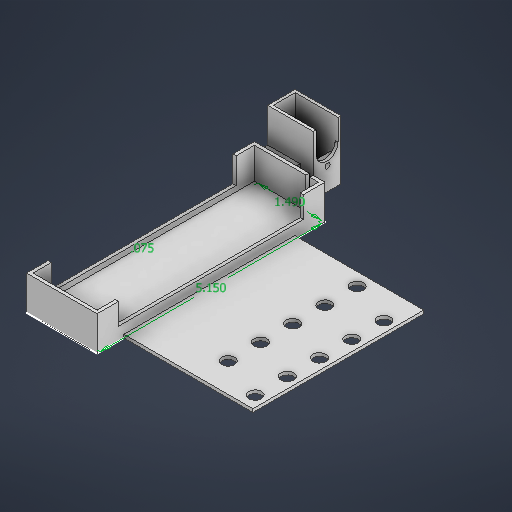
# Autodesk Inventor part: HarmonicaFrame2
Saved by Autodesk Inventor 2026.2 (Build 302298010, 298A)
## iProperties
Created: 2026-03-08
Part Number: HarmonicaFrame2
Material: Generic
Document SubType Name: Modeling
Designer: david
Density: 1 g/cm^3
Appearance: Default
Author: david
Autodesk Inventor part; units mm, degrees
ref_plane "YZ Plane" through (0, 0, 0) normal (1, 0, 0) x (0, 1, 0)
ref_plane "XZ Plane" through (0, 0, 0) normal (0, 1, 0) x (-1, 0, 0)
ref_plane "XY Plane" through (0, 0, 0) normal (0, 0, 1) x (1, 0, 0)
sketch "Sketch1" plane through (0, 0, 0) normal (0, 1, 0) x (-1, 0, 0)
  line L0 (18.923, 65.405) -> (-18.923, 65.405)
  line L1 (-18.923, 65.405) -> (-18.923, -65.405)
  line L2 (-18.923, -65.405) -> (18.923, -65.405)
  line L3 (18.923, -65.405) -> (18.923, 65.405)
  line L4 (18.923, 65.405) -> (-18.923, -65.405) construction
  line L5 (-18.923, 65.405) -> (18.923, -65.405) construction
  line L6 (20.828, 67.31) -> (-20.828, 67.31)
  line L7 (-20.828, 67.31) -> (-20.828, -67.31)
  line L8 (-20.828, -67.31) -> (20.828, -67.31)
  line L9 (20.828, -67.31) -> (20.828, 67.31)
  point P0 (0, 0)
  dimension "d0" = 37.846
  dimension "d1" = 130.81
  dimension "d2" = 1.905
  constraints: 20 end point, 4 parallel, 2 midpoint, 2 perpendicular, 1 horizontal, 3 other
  measures "d0" distance of L2.end L1.end
  measures "d1" distance of L1.end L0.end
  measures "d2" distance between parallel lines of L3 L9
extrude "Extrusion1" add sketch "Sketch1" along normal blind 20.32
extrude "Extrusion2" add sketch "Sketch1" along normal blind 1.905 contours L3 L2 L1 L0
sketch "Sketch2" plane through (20.828, 0, 67.31) normal (1, 0, 0) x (0, 0, -1)
  line L0 (12.7, 20.32) -> (121.92, 20.32)
  line L1 (121.92, 20.32) -> (121.92, 7.62)
  line L2 (121.92, 7.62) -> (12.7, 7.62)
  line L3 (12.7, 7.62) -> (12.7, 20.32)
  line L4 (0, 0) -> (0, 20.32) projected
  line L5 (134.62, 0) -> (134.62, 20.32) projected
  line L6 (0, 20.32) -> (134.62, 20.32) projected
  line L7 (0, 0) -> (134.62, 0) projected
  point P0 (67.31, 0)
  dimension "d7" = 12.7
  dimension "d8" = 12.7
  dimension "d9" = 7.62
  constraints: 8 end point, 2 parallel, 1 collinear, 1 horizontal, 1 perpendicular
  measures "d7" distance between parallel lines of L4 L3
  measures "d8" distance between parallel lines of L5 L1
  measures "d9" distance between parallel lines of L7 L2
extrude "Extrusion3" cut sketch "Sketch2" against normal blind 1.905 contours L0 L1 L2 L3
sketch "Sketch3" plane through (-20.828, 0, -67.31) normal (-1, 0, 0) x (0, 0, 1)
  line L0 (12.7, 20.32) -> (121.92, 20.32)
  line L1 (121.92, 20.32) -> (121.92, 5.08)
  line L2 (121.92, 5.08) -> (12.7, 5.08)
  line L3 (12.7, 5.08) -> (12.7, 20.32)
  line L4 (0, 20.32) -> (134.62, 20.32) projected
  line L5 (0, 0) -> (0, 20.32) projected
  line L6 (134.62, 0) -> (134.62, 20.32) projected
  line L7 (0, 0) -> (134.62, 0) projected
  point P0 (67.31, 0)
  dimension "d12" = 12.7
  dimension "d13" = 12.7
  dimension "d14" = 5.08
  constraints: 8 end point, 2 parallel, 1 collinear, 1 horizontal, 1 perpendicular
  measures "d12" distance between parallel lines of L5 L3
  measures "d13" distance between parallel lines of L6 L1
  measures "d14" distance between parallel lines of L7 L2
extrude "Extrusion4" cut sketch "Sketch3" against normal blind 1.905 contours L0 L1 L2 L3
sketch "Sketch4" plane through (0, 20.32, 0) normal (0, 1, 0) x (1, 0, 0)
  line L0 (20.828, 67.31) -> (-20.828, 67.31) projected
  line L1 (-18.923, 65.405) -> (18.923, 65.405) projected
  line L2 (13.843, 67.31) -> (11.557, 67.31)
  line L3 (11.557, 67.31) -> (11.557, 65.405)
  line L4 (11.557, 65.405) -> (13.843, 65.405)
  line L5 (13.843, 65.405) -> (13.843, 67.31)
  line L6 (18.923, 65.405) -> (18.923, 54.61) projected
  line L7 (-18.923, 54.61) -> (-18.923, 65.405) projected
  point P0 (0, 0)
  dimension "d17" = 5.08
  dimension "d18" = 30.48
  constraints: 8 end point, 2 parallel, 2 point on line, 1 horizontal, 1 perpendicular
  measures "d17" distance between parallel lines of L6 L5
  measures "d18" distance between parallel lines of L7 L3
extrude "Extrusion5" cut sketch "Sketch4" against normal up to surface (18.415 mm away)
sketch "Sketch5" plane through (20.828, 0, -67.31) normal (0, 0, -1) x (-1, 0, 0)
  line L0 (0, 0) -> (41.656, 0) projected
  line L1 (0, 0) -> (41.656, 0)
  line L2 (41.656, 0) -> (41.656, 1.905)
  line L3 (41.656, 1.905) -> (0, 1.905)
  line L4 (0, 1.905) -> (0, 0)
  line L5 (9.271, 1.905) -> (6.985, 1.905) projected
  line L6 (41.656, 0) -> (41.656, 20.32) projected
  point P0 (20.828, 0)
  constraints: 8 end point, 2 collinear, 2 parallel, 1 horizontal, 1 perpendicular
extrude "Extrusion6" add sketch "Sketch5" along normal blind 24.13
sketch "Sketch6" plane through (0, 1.905, 0) normal (0, 1, 0) x (1, 0, 0)
  line L0 (-19.177, 76.835) -> (4.445, 76.835)
  line L1 (4.445, 76.835) -> (4.445, 89.789)
  line L2 (4.445, 89.789) -> (-19.177, 89.789)
  line L3 (-19.177, 89.789) -> (-19.177, 76.835)
  line L4 (18.923, 65.405) -> (18.923, 54.61) projected
  line L5 (11.557, 67.31) -> (-20.828, 67.31) projected
  line L6 (-20.828, 75.184) -> (6.096, 75.184)
  line L7 (6.096, 75.184) -> (6.096, 91.44)
  line L8 (6.096, 91.44) -> (-20.828, 91.44)
  line L9 (-20.828, 91.44) -> (-20.828, 75.184)
  line L10 (-20.828, 91.44) -> (20.828, 91.44) projected
  line L11 (-20.828, 67.31) -> (-20.828, 91.44) projected
  line L12 (-18.923, 65.405) -> (11.557, 65.405) projected
  point P0 (0, 0)
  dimension "d24" = 12.954
  dimension "d26" = 23.622
  dimension "d32" = 11.43
  constraints: 16 end point, 4 parallel, 2 collinear, 2 perpendicular, 1 horizontal, 3 other
  measures "d24" distance between parallel lines of L2 L0
  measures "d26" distance between parallel lines of L1 L3
  measures "d32" distance between parallel lines of L12 L0
extrude "Extrusion7" add sketch "Sketch6" along normal blind 33.02
sketch "Sketch8" plane through (4.445, 1.905, -89.789) normal (-1, 0, 0) x (0, 0, 1)
  circle A0 centre (6.477, 20.32) radius 6.477
  line L0 (0, 0) -> (0, 33.02) projected
  line L1 (12.954, 0) -> (12.954, 33.02) projected
  line L2 (0, 0) -> (12.954, 0) projected
  line L3 (12.954, 20.32) -> (12.954, 33.02)
  line L4 (0, 33.02) -> (0, 20.32)
  line L5 (12.954, 33.02) -> (0, 33.02)
  line L6 (12.954, 20.32) -> (12.954, 33.02)
  line L7 (0, 33.02) -> (0, 20.32)
  point P0 (89.789, -1.905)
  dimension "d29" = 20.32
  constraints: 10 end point, 5 tangent, 2 collinear, 2 point on circle, 2 point on line, 1 centre point, 1 parallel, 1 perpendicular
  measures "d29" distance from line of L2 A0.centre
extrude "Extrusion8" cut sketch "Sketch8" against normal blind 33.02 contours A0 | A0 L0 L5 L1
sketch "Sketch10" plane through (4.445, 1.905, -89.789) normal (-1, 0, 0) x (0, 0, 1)
  line L0 (-1.651, 0) -> (14.605, 0) projected
  line L1 (-1.651, 0) -> (-1.651, 33.02) projected
  line L2 (14.605, 0) -> (-1.651, 0)
  line L3 (-1.651, 0) -> (-1.651, 13.208)
  line L4 (-1.651, 13.208) -> (14.605, 13.208)
  line L5 (14.605, 13.208) -> (14.605, 0)
  arc A0 (0, 20.32) -> (12.954, 20.32) centre (6.477, 20.32) ccw projected
  point P0 (89.789, -1.905)
  point P1 (6.477, 13.843)
  point P2 (6.477, 13.208)
  dimension "d37" = 0.635
  constraints: 8 end point, 2 parallel, 1 horizontal, 1 midpoint, 1 perpendicular, 1 point on circle, 1 point on line
  measures "d37" distance of point (6.477, 13.843) point (6.477, 13.208)
extrude "Extrusion10" add sketch "Sketch10" along normal blind 3.048
sketch "Sketch9" plane through (6.096, 1.905, -75.184) normal (1, 0, 0) x (0, 0, -1)
  arc A0 (1.651, 20.32) -> (14.605, 20.32) centre (8.128, 20.32) ccw projected
  circle A1 centre (8.372, 11.303) radius 1.524
  point P0 (-75.184, -1.905)
  point P1 (8.128, 13.843)
  dimension "d33" = 2.54
  dimension "d34" = 3.048
  constraints: 1 centre point, 1 coincident, 1 point on circle
  measures "d33" vertical distance of point (8.372, 11.303) point (8.128, 13.843)
  measures "d34" diameter of A1
extrude "Extrusion9" cut sketch "Sketch9" against normal up to surface (25.273 mm away)
sketch "Sketch11" plane through (20.828, 0, 67.31) normal (1, 0, 0) x (0, 0, -1)
  line L0 (134.62, 1.905) -> (158.75, 1.905) projected
  line L1 (0, 0) -> (158.75, 0)
  line L2 (158.75, 0) -> (158.75, 1.905)
  line L3 (158.75, 1.905) -> (0, 1.905)
  line L4 (0, 1.905) -> (0, 0)
  point P0 (67.31, 0)
  constraints: 8 end point, 2 parallel, 1 horizontal, 1 perpendicular
extrude "Extrusion11" add sketch "Sketch11" along normal blind 76.2
sketch "Sketch12" plane through (0, 1.905, 0) normal (0, 1, 0) x (1, 0, 0)
  circle A0 centre (90.678, -43.815) radius 3.81
  line L0 (20.828, 54.61) -> (20.828, -54.61) projected
  line L1 (18.923, -65.405) -> (-18.923, -65.405) projected
  line L2 (20.828, -51.435) -> (97.028, -51.435)
  line L3 (97.028, 91.44) -> (97.028, -67.31) projected
  line L4 (97.028, -67.31) -> (20.828, -67.31)
  line L5 (20.828, -67.31) -> (20.828, -51.435)
  line L6 (97.028, -36.195) -> (20.828, -36.195)
  line L7 (-20.828, 91.44) -> (97.028, 91.44) projected
  line L8 (20.828, 91.44) -> (97.028, 91.44)
  line L9 (97.028, 91.44) -> (97.028, -36.195)
  line L10 (20.828, -36.195) -> (97.028, -36.195)
  line L11 (97.028, -36.195) -> (97.028, 91.44)
  line L12 (97.028, 91.44) -> (20.828, 91.44)
  line L13 (20.828, 91.44) -> (20.828, -36.195)
  line L14 (6.096, 91.44) -> (97.028, 91.44)
  line L15 (97.028, 91.44) -> (97.028, 67.31)
  line L16 (6.096, 67.31) -> (6.096, 91.44)
  line L17 (6.096, 89.789) -> (6.096, 91.44) projected
  line L18 (20.828, 67.31) -> (13.843, 67.31) projected
  circle A1 centre (65.278, -34.29) radius 3.81
  circle A2 centre (90.678, -24.765) radius 3.81
  circle A3 centre (90.678, -5.715) radius 3.81
  circle A4 centre (90.678, 13.335) radius 3.81
  circle A5 centre (90.678, 32.385) radius 3.81
  circle A6 centre (65.278, -15.24) radius 3.81
  circle A7 centre (65.278, 3.81) radius 3.81
  circle A8 centre (65.278, 22.86) radius 3.81
  circle A9 centre (65.278, 41.91) radius 3.81
  line L19 (20.828, 91.44) -> (97.028, 91.44)
  line L20 (97.028, 91.44) -> (97.028, 49.53)
  line L21 (97.028, 49.53) -> (20.828, 49.53)
  line L22 (20.828, 49.53) -> (20.828, 91.44)
  line L23 (6.096, 67.31) -> (20.828, 67.31)
  line L24 (20.828, 67.31) -> (20.828, 91.44)
  line L25 (20.828, 91.44) -> (6.096, 91.44)
  line L26 (6.096, 91.44) -> (6.096, 67.31)
  point P0 (0, 0)
  point P1 (97.028, -36.195)
  point P2 (20.828, -54.61)
  point P3 (6.096, 90.5705)
  point P4 (5.715, 89.789)
  point P5 (20.828, 49.53)
  dimension "d42" = 7.62
  dimension "d44" = 21.59
  dimension "d45" = 7.62
  dimension "d46" = 7.62
  dimension "d59" = 7.62
  dimension "d76" = 69.85
  dimension "d79" = 19.05
  dimension "d84" = 9.525
  dimension "d87" = 19.05
  dimension "d92" = 25.4
  dimension "d93" = 7.62
  constraints: 40 end point, 10 centre point, 8 point on line, 6 horizontal, 6 parallel, 6 perpendicular, 3 vertical, 2 collinear, 22 other
  measures "d42" diameter of A0
  measures "d44" distance from line of L1 A0.centre
  measures "d45" distance from line of A0.centre L2
  measures "d46" distance from line of A0.centre L6
  measures "d59" diameter of A1
  measures "d76" distance from line of L0 A0.centre
  measures "d79" distance of A0.centre A2.centre
  measures "d84" vertical distance of A0.centre A1.centre
  measures "d87" distance of A1.centre A6.centre
  measures "d92" horizontal distance of A0.centre A1.centre
  measures "d93" distance from line of A9.centre L21
extrude "Extrusion12" cut sketch "Sketch12" against normal blind 57.15 contours A0 | L13 L7 L3 L21 L0 | L18 L23 L16 L7 L13 | L2 L3 L4 L5 L0 | A1 L6 | L6 A1 | A2 | A3 | A4 | A5 | A6 | A7 | A8 | A9
sketch "Sketch13" plane through (0, 1.905, 0) normal (0, 1, 0) x (1, 0, 0)
  line L0 (11.557, 67.31) -> (-20.828, 67.31) projected
  line L1 (-20.828, 75.184) -> (6.096, 75.184) projected
  line L2 (-13.208, 67.31) -> (-1.524, 67.31)
  line L3 (-1.524, 67.31) -> (-1.524, 75.184)
  line L4 (-1.524, 75.184) -> (-13.208, 75.184)
  line L5 (-13.208, 75.184) -> (-13.208, 67.31)
  line L6 (-20.828, 67.31) -> (-20.828, 75.184) projected
  line L7 (6.096, 91.44) -> (6.096, 75.184) projected
  point P0 (0, 0)
  point P1 (-20.828, 71.247)
  point P2 (-13.208, 71.247)
  point P3 (6.096, 67.31)
  point P4 (-1.524, 67.31)
  point P5 (-13.208, 75.184)
  point P6 (-1.524, 67.31)
  dimension "d49" = 7.62
  dimension "d50" = 7.62
  constraints: 8 end point, 2 midpoint, 2 parallel, 2 point on line, 1 horizontal, 1 perpendicular
  measures "d49" distance of point (-20.828, 71.247) point (-13.208, 71.247)
  measures "d50" distance between parallel lines of L7 L3
extrude "Extrusion13" add sketch "Sketch13" along normal blind 12.7
sketch "Sketch15" plane through (-19.177, 1.905, -76.835) normal (1, 0, 0) x (0, 0, -1)
  line L0 (0, 0) -> (12.954, 0)
  line L1 (12.954, 0) -> (12.954, 6.35)
  line L2 (12.954, 6.35) -> (0, 6.35)
  line L3 (0, 6.35) -> (0, 0)
  line L4 (-144.145, -1.905) -> (14.605, -1.905) projected
  line L5 (14.605, -1.905) -> (14.605, 33.02) projected
  point P0 (-76.835, -1.905)
  dimension "d94" = 12.954
  dimension "d95" = 6.35
  dimension "d96" = 1.905
  dimension "d97" = 1.651
  constraints: 8 end point, 2 parallel, 1 horizontal, 1 perpendicular
  measures "d94" distance of L2.end L1.end
  measures "d95" distance of L1.end L0.end
  measures "d96" distance between parallel lines of L4 L0
  measures "d97" distance between parallel lines of L5 L1
extrude "Extrusion14" cut sketch "Sketch15" against normal blind 57.15
body "Solid1"
